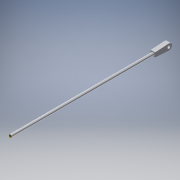
# Autodesk Inventor part: Rod
Saved by Autodesk Inventor 2016 (Build 200138000, 138)
## iProperties
Created: 2015-05-18
Part Number: Rod
Material: Generic
Document SubType Name: Modeling
Designer: Andy
Density: 4.17152 g/cm^3
Appearance: Default
Mass: 125 g
Surface Area: 143.864 cm^2
Volume: 29.9651 cm^3
Author: Andy
Autodesk Inventor part; units mm, degrees
ref_plane "YZ Plane" through (0, 0, 0) normal (1, 0, 0) x (0, 1, 0)
ref_plane "XZ Plane" through (0, 0, 0) normal (0, 1, 0) x (-1, 0, 0)
ref_plane "XY Plane" through (0, 0, 0) normal (0, 0, 1) x (1, 0, 0)
sketch "Sketch1" plane through (0, 0, 0) normal (0, 1, 0) x (-1, 0, 0)
  circle A0 centre (0, 0) radius 4
  dimension "d0" = 8
  constraints: 1 centre point, 1 coincident
  measures "d0" diameter of A0
extrude "Extrusion1" add sketch "Sketch1" along normal blind 433.3875
sketch "Sketch2" plane through (0, 433.3875, 0) normal (0, 1, 0) x (1, 0, 0)
  circle A0 centre (0, 0) radius 4 projected
  line L0 (6.5, -6.5) -> (-6.5, -6.5)
  line L1 (-6.5, -6.5) -> (-6.5, 6.5)
  line L2 (-6.5, 6.5) -> (6.5, 6.5)
  line L3 (6.5, 6.5) -> (6.5, -6.5)
  line L4 (6.5, -6.5) -> (-6.5, 6.5) construction
  line L5 (-6.5, -6.5) -> (6.5, 6.5) construction
  dimension "d3" = 13
  dimension "d4" = 13
  constraints: 12 end point, 2 midpoint, 2 parallel, 1 horizontal, 1 perpendicular
  measures "d3" distance of L1.end L2.end
  measures "d4" distance of L0.end L1.end
extrude "Extrusion2" add sketch "Sketch2" along normal blind 41 contours A0 | L0 L1 L2 L3
sketch "Sketch3" plane through (-6.5, 433.3875, -6.5) normal (-1, 0, 0) x (0, 0, 1)
  line L0 (13, 0) -> (13, 41) projected
  line L1 (0, 0) -> (0, 41) projected
  line L2 (13, 41) -> (0, 41) projected
  arc A0 (15.4333, 39.9065) -> (-2.4333, 39.9065) centre (6.5, 41) ccw
  line L3 (13, 0) -> (15.5, 41)
  line L4 (0, 0) -> (-2.5, 41)
  point P0 (6.5, -433.3875)
  dimension "d7" = 18
  constraints: 4 end point, 4 point on circle, 2 point on line, 1 centre point, 1 midpoint
  measures "d7" diameter of A0
extrude "Extrusion3" add sketch "Sketch3" against normal blind 13 contours L0 L2 L1 L4 A0 L3
sketch "Sketch4" plane through (-6.5, 474.3875, 0) normal (-1, 0, 0) x (0, 0, 1)
  arc A0 (9, 0) -> (-9, 0) centre (0, 0) ccw projected
  circle A1 centre (0, 0) radius 4.5
  point P0 (0, -474.3875)
  dimension "d11" = 9
  constraints: 1 centre point, 1 coincident
  measures "d11" diameter of A1
extrude "Extrusion4" cut sketch "Sketch4" against normal blind 15
sketch "Sketch5" plane through (6.5, 433.3875, 6.5) normal (1, 0, 0) x (0, 0, -1)
  line L0 (13, 0) -> (15.5, 41) projected
  line L1 (13, 0) -> (14.2173, 19.9629)
  circle A0 centre (6.5, 41) radius 4.5 projected
  line L2 (14.2173, 19.9629) -> (6.5, 41)
  line L3 (14.2173, 19.9629) -> (6.5, 41)
  line L4 (6.5, 41) -> (7.4388, 41.3444)
  line L5 (7.4388, 41.3444) -> (15.1561, 20.3073)
  line L6 (15.1561, 20.3073) -> (14.2173, 19.9629)
  point P0 (6.5, -433.3875)
  dimension "d25" = 20
  dimension "d26" = 1
  constraints: 12 end point, 3 equal length, 1 perpendicular, 1 point on line
  measures "d25" distance of L0.start L1.end
  measures "d26" distance of L2.end L4.end
extrude "Extrusion5" [suppressed]
sketch "Sketch6" plane through (6.5, 433.3875, -6.5) normal (0, -0.0609, -0.9981) x (-1, 0, 0)
  line L0 (13, 20) -> (0, 20) projected
  line L1 (13, 0) -> (0, 0) projected
  line L2 (6.5, 0) -> (6.5, 32)
  point P0 (6.5, -432.9797)
  dimension "d29" = 32
  constraints: 2 end point, 1 midpoint, 1 perpendicular
  measures "d29" distance of L2.start L2.end
hole "Hole2" [suppressed]
thread "Thread2" size "M3x0.5" class "6H" standard "ANSI Metric M Profile" full length
sketch "Sketch7" plane through (0, 0, 0) normal (1, 0, 0) x (0, 1, 0)
  line L0 (0, 0) -> (12.7, 0)
  line L1 (0, 0) -> (-16.3, 0)
  line L2 (0, 0) -> (-1.8, 0)
  arc A0 (-1.8, 14.5) -> (-1.8, -14.5) centre (-1.8, 0) ccw
  line L3 (-1.8, 14.5) -> (-1.8, -14.5)
  dimension "d41" = 12.7
  dimension "d43" = 1.8
  constraints: 8 end point, 2 horizontal, 2 point on circle, 1 centre point, 1 coincident, 1 midpoint, 1 point on line, 1 vertical
  measures "d41" distance of L0.start L0.end
  measures "d43" distance of L0.start L2.end
revolve "Revolution1" cut sketch "Sketch7" angle 360 about axis through (0, -1.8, 14.5) along (0, 0, -1)
body "Solid1"
